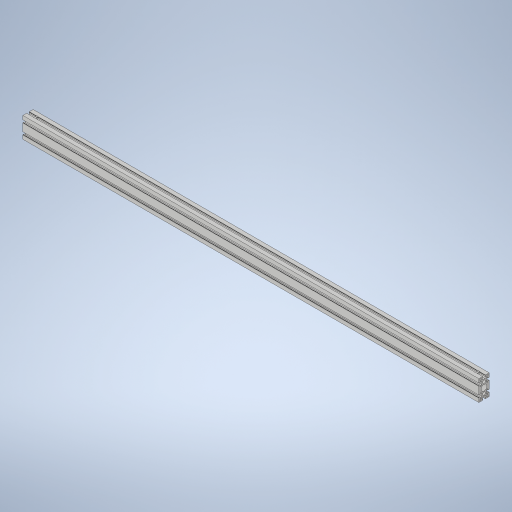
# Autodesk Inventor part: Perfil 45X90x1990
Saved by Autodesk Inventor 2024.2 (Build 282272000, 272)
## iProperties
Created: 2024-05-14
Part Number: Perfil 45X90x1990
Material: Genérico
Document SubType Name: Modeling
Designer: lugomez
Density: 1 g/cm^3
Appearance: Por defecto
Author: lugomez
Autodesk Inventor part; units mm, degrees
ref_plane "YZ Plane" through (0, 0, 0) normal (1, 0, 0) x (0, 1, 0)
ref_plane "XZ Plane" through (0, 0, 0) normal (0, 1, 0) x (-1, 0, 0)
ref_plane "XY Plane" through (0, 0, 0) normal (0, 0, 1) x (1, 0, 0)
sketch "Boceto1" plane through (0, 0, 0) normal (1, 0, 0) x (0, 1, 0)
  circle A0 centre (0, 0) radius 12.5
  line L0 (0, 22.5) -> (16.5, 22.5)
  line L1 (16.5, 22.5) -> (16.5, 21)
  line L2 (16.5, 21) -> (17.5, 21)
  line L3 (17.5, 21) -> (17.5, 16.5)
  line L4 (17.5, 16.5) -> (12.5, 16.5)
  line L5 (12.5, 16.5) -> (12.5, 12.5)
  line L6 (12.5, 12.5) -> (17.5, 10)
  line L7 (17.5, 10) -> (27.5, 10)
  line L8 (32.5, 12.5) -> (32.5, 16.5)
  line L9 (32.5, 16.5) -> (27.5, 16.5)
  line L10 (27.5, 16.5) -> (27.5, 21)
  line L11 (27.5, 21) -> (28.5, 21)
  line L12 (28.5, 21) -> (28.5, 22.5)
  line L13 (28.5, 22.5) -> (45, 22.5)
  line L14 (45, 22.5) -> (45, 6)
  line L15 (45, 6) -> (43.5, 6)
  line L16 (43.5, 6) -> (43.5, 5)
  line L17 (43.5, 5) -> (39, 5)
  line L18 (32.5, 12.5) -> (27.5, 10)
  line L19 (0, 0) -> (0, 104.1484) construction
  line L20 (0, 0) -> (99.9828, 0) construction
  line L21 (39, 5) -> (39, 10)
  line L22 (39, 10) -> (35, 10)
  line L23 (35, 10) -> (32.5, 5)
  line L24 (32.5, 5) -> (32.5, 0)
  circle A1 centre (22.5, 0) radius 6
  circle A2 centre (39, 16.5) radius 3
  line L25 (0, 0) -> (68.012, 0) construction
  line L26 (0, -22.5) -> (16.5, -22.5)
  line L27 (16.5, -22.5) -> (16.5, -21)
  line L28 (16.5, -21) -> (17.5, -21)
  line L29 (17.5, -21) -> (17.5, -16.5)
  line L30 (17.5, -16.5) -> (12.5, -16.5)
  line L31 (12.5, -16.5) -> (12.5, -12.5)
  line L32 (12.5, -12.5) -> (17.5, -10)
  line L33 (17.5, -10) -> (27.5, -10)
  line L34 (32.5, -12.5) -> (32.5, -16.5)
  line L35 (32.5, -16.5) -> (27.5, -16.5)
  line L36 (27.5, -16.5) -> (27.5, -21)
  line L37 (27.5, -21) -> (28.5, -21)
  line L38 (28.5, -21) -> (28.5, -22.5)
  line L39 (28.5, -22.5) -> (45, -22.5)
  line L40 (45, -22.5) -> (45, -6)
  line L41 (45, -6) -> (43.5, -6)
  line L42 (43.5, -6) -> (43.5, -5)
  line L43 (43.5, -5) -> (39, -5)
  line L44 (32.5, -12.5) -> (27.5, -10)
  line L45 (39, -5) -> (39, -10)
  line L46 (39, -10) -> (35, -10)
  line L47 (35, -10) -> (32.5, -5)
  line L48 (32.5, -5) -> (32.5, 0)
  circle A3 centre (39, -16.5) radius 3
  line L49 (0, 22.5) -> (-16.5, 22.5)
  line L50 (-16.5, 22.5) -> (-16.5, 21)
  line L51 (-16.5, 21) -> (-17.5, 21)
  line L52 (-17.5, 21) -> (-17.5, 16.5)
  line L53 (-17.5, 16.5) -> (-12.5, 16.5)
  line L54 (-12.5, 16.5) -> (-12.5, 12.5)
  line L55 (-12.5, 12.5) -> (-17.5, 10)
  line L56 (-17.5, 10) -> (-27.5, 10)
  line L57 (-32.5, 12.5) -> (-32.5, 16.5)
  line L58 (-32.5, 16.5) -> (-27.5, 16.5)
  line L59 (-27.5, 16.5) -> (-27.5, 21)
  line L60 (-27.5, 21) -> (-28.5, 21)
  line L61 (-28.5, 21) -> (-28.5, 22.5)
  line L62 (-28.5, 22.5) -> (-45, 22.5)
  line L63 (-45, 22.5) -> (-45, 6)
  line L64 (-45, 6) -> (-43.5, 6)
  line L65 (-43.5, 6) -> (-43.5, 5)
  line L66 (-43.5, 5) -> (-39, 5)
  line L67 (-32.5, 12.5) -> (-27.5, 10)
  line L68 (-39, 5) -> (-39, 10)
  line L69 (-39, 10) -> (-35, 10)
  line L70 (-35, 10) -> (-32.5, 5)
  line L71 (-32.5, 5) -> (-32.5, 0)
  circle A4 centre (-22.5, 0) radius 6
  circle A5 centre (-39, 16.5) radius 3
  line L72 (-43.5, -6) -> (-43.5, -5)
  line L73 (-45, -6) -> (-43.5, -6)
  line L74 (-32.5, -12.5) -> (-32.5, -16.5)
  line L75 (-35, -10) -> (-32.5, -5)
  line L76 (-39, -5) -> (-39, -10)
  line L77 (-39, -10) -> (-35, -10)
  line L78 (-32.5, -12.5) -> (-27.5, -10)
  line L79 (-45, -22.5) -> (-45, -6)
  circle A6 centre (-39, -16.5) radius 3
  line L80 (-28.5, -22.5) -> (-45, -22.5)
  line L81 (-27.5, -16.5) -> (-27.5, -21)
  line L82 (-27.5, -21) -> (-28.5, -21)
  line L83 (-28.5, -21) -> (-28.5, -22.5)
  line L84 (-32.5, -16.5) -> (-27.5, -16.5)
  line L85 (-43.5, -5) -> (-39, -5)
  line L86 (-32.5, -5) -> (-32.5, 0)
  line L87 (-17.5, -10) -> (-27.5, -10)
  line L88 (0, -22.5) -> (-16.5, -22.5)
  line L89 (-16.5, -22.5) -> (-16.5, -21)
  line L90 (-16.5, -21) -> (-17.5, -21)
  line L91 (-17.5, -21) -> (-17.5, -16.5)
  line L92 (-17.5, -16.5) -> (-12.5, -16.5)
  line L93 (-12.5, -16.5) -> (-12.5, -12.5)
  line L94 (-12.5, -12.5) -> (-17.5, -10)
  point P0 (22.5, 10)
  point P1 (22.5, -10)
  point P2 (-22.5, 10)
  point P3 (-22.5, -10)
  dimension "d0" = 25
  dimension "d1" = 22.5
  dimension "d3" = 20
  dimension "d4" = 1.5
  dimension "d5" = 1.5
  dimension "d6" = 10
  dimension "d7" = 12
  dimension "d8" = 12.5
  dimension "d9" = 22.5
  dimension "d10" = 5
  dimension "d11" = 6
  dimension "d12" = 10
  dimension "d13" = 6
  dimension "d14" = 4
  dimension "d15" = 5
  dimension "d17" = 6
  dimension "d18" = 45
  dimension "d20" = 10
  dimension "d21" = 4
  dimension "d22" = 12.5
  dimension "d23" = 6
  dimension "d24" = 12
  dimension "d25" = 22.5
  dimension "d26" = 6
  dimension "d27" = 39
  dimension "d28" = 16.5
  constraints: 190 end point, 75 symmetric about line, 23 point on line, 12 perpendicular, 7 centre point, 3 horizontal alignment, 3 vertical, 2 horizontal, 2 parallel, 1 coincident, 1 collinear, 1 midpoint, 1 vertical alignment, 4 other
  measures "d0" diameter of A0
  measures "d1" distance from line of point (0, 0) L0
  measures "d3" distance between parallel lines of L5 L8
  measures "d4" distance between parallel lines of L0 L2
  measures "d5" distance between parallel lines of L14 L16
  measures "d6" distance between parallel lines of L10 L3
  measures "d7" distance between parallel lines of L1 L12
  measures "d8" distance between parallel lines of L0 L7
  measures "d9" horizontal distance of point (22.5, 10) point (0, 0)
  measures "d10" distance from line of point (22.5, 10) L10
  measures "d11" distance from line of point (22.5, 10) L12
  measures "d12" distance from line of point (22.5, 10) L5
  measures "d13" distance between parallel lines of L0 L4
  measures "d14" distance of L4.end L5.end
  measures "d15" distance between parallel lines of L20 L17
  measures "d17" distance between parallel lines of L20 L15
  measures "d18" distance from line of point (0, 0) L14
  measures "d20" distance between parallel lines of L20 L22
  measures "d21" distance of L21.end L22.end
  measures "d22" distance between parallel lines of L14 L24
  measures "d23" distance between parallel lines of L14 L21
  measures "d24" diameter of A1
  measures "d25" distance of point (0, 0) A1.centre
  measures "d26" diameter of A2
  measures "d27" horizontal distance of A2.centre point (0, 0)
  measures "d28" vertical distance of point (0, 0) A2.centre
extrude "Derecha 1590" add sketch "Boceto1" along normal blind 1990
sketch "Boceto2" plane through (0, 45, -6) normal (0, 1, 0) x (1, 0, 0)
  line L0 (1990, -1) -> (1990, -11) projected
  line L1 (0, -1) -> (0, -11) projected
  point P0 (0, -6)
  point P1 (32, -6)
  point P2 (1958, -6)
  point P3 (1990, -6)
  dimension "d31" = 32
  dimension "d32" = 32
  constraints: 2 horizontal alignment, 1 midpoint
  measures "d31" distance from line of L0 point (1958, -6)
  measures "d32" distance from line of point (32, -6) L1
hole "Agujero1" at (32, 45, 0) at (1958, 45, 0) direction (0, -1, 0) diameter 15.1 depth 30.5 tip angle 118
sketch "Boceto3" plane through (0, -45, -22.5) normal (0, -1, 0) x (1, 0, 0)
  line L0 (1990, 27.5) -> (1990, 17.5) projected
  point P0 (0, 22.5)
  point P1 (32, 22.5)
  point P2 (1958, 22.5)
  point P3 (1990, 22.5)
  dimension "d40" = 32
  dimension "d41" = 32
  constraints: 2 horizontal alignment, 1 midpoint
  measures "d40" distance of point (32, 22.5) point (0, 22.5)
  measures "d41" distance from line of point (1958, 22.5) L0
hole "Agujero2" at (32, -45, 0) at (1958, -45, 0) direction (0, 1, 0) diameter 15.1 depth 30.5 tip angle 118
equation "\"d5\" = d4"
equation "\"d10\" = 0.5 * d6"
equation "\"d11\" = 0.5 * d7"
equation "\"d12\" = 0.5 * d3"
equation "\"d15\" = d10"
equation "\"d17\" = d11"
equation "\"d20\" = d12"
equation "\"d21\" = d14"
equation "\"d23\" = d13"
